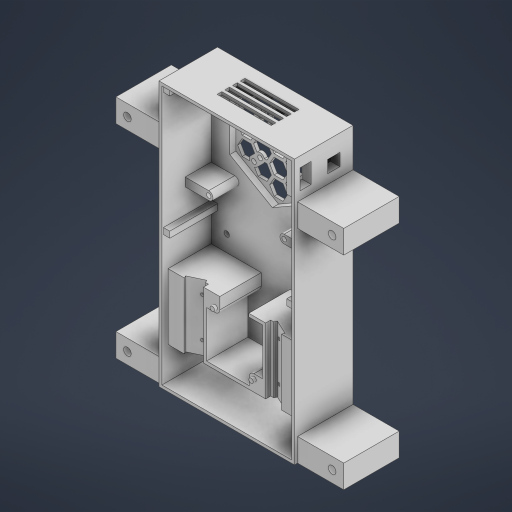
# Autodesk Inventor part: PrimaryCase
Saved by Autodesk Inventor 2023 (Build 270158000, 158)
## iProperties
Created: 2023-12-04
Part Number: PrimaryCase
Material: Generic
Document SubType Name: Modeling
Designer: FizzyApple12
Density: 1 g/cm^3
Appearance: Default
Author: FizzyApple12
Autodesk Inventor part; units mm, degrees
ref_plane "YZ Plane" through (0, 0, 0) normal (1, 0, 0) x (0, 1, 0)
ref_plane "XZ Plane" through (0, 0, 0) normal (0, 1, 0) x (-1, 0, 0)
ref_plane "XY Plane" through (0, 0, 0) normal (0, 0, 1) x (1, 0, 0)
sketch "Sketch1" plane through (0, 0, 0) normal (0, 0, 1) x (1, 0, 0)
  line L0 (0, 0) -> (84, 0)
  line L1 (84, 0) -> (84, -84)
  line L2 (84, -84) -> (0, -84)
  line L3 (0, -84) -> (0, 0)
  line L4 (0, 84) -> (84, 84)
  line L5 (84, 84) -> (84, 0)
  line L6 (84, 0) -> (0, 0) construction
  line L7 (0, 0) -> (0, 84)
  line L8 (-2, 86) -> (86, 86)
  line L9 (86, 86) -> (86, -86)
  line L10 (86, -86) -> (-2, -86)
  line L11 (-2, -86) -> (-2, 86)
  line L12 (-2, 86) -> (86, -86) construction
  line L13 (17, 67) -> (67, 67)
  line L14 (67, 67) -> (67, 17)
  line L15 (67, 17) -> (17, 17)
  line L16 (17, 17) -> (17, 67)
  line L17 (0, 0) -> (84, 84) construction
  line L18 (17, 67) -> (67, 17) construction
  line L19 (0, 2) -> (84, 2)
  point P0 (42, 0)
  point P1 (42, 42)
  point P2 (84, 0)
  dimension "d0" = 84
  dimension "d1" = 84
  dimension "d2" = 84
  dimension "d3" = 84
  dimension "d4" = 88
  dimension "d5" = 172
  dimension "d6" = 50
  dimension "d7" = 50
  dimension "d20" = 2
  constraints: 40 end point, 8 parallel, 5 perpendicular, 4 horizontal, 4 midpoint, 2 point on line
  measures "d0" distance of L1.end L2.end
  measures "d1" distance of L0.end L1.end
  measures "d2" distance of L0.start L5.end
  measures "d3" distance of L4.end L5.end
  measures "d4" distance of L9.end L10.end
  measures "d5" distance of L8.end L9.end
  measures "d6" distance of L14.end L15.end
  measures "d7" distance of L13.end L14.end
  measures "d20" distance between parallel lines of L0 L19
extrude "Extrusion1" add sketch "Sketch1" against normal blind 40 contours L8 L9 L10 L11
sketch "Sketch3" plane through (0, 0, -40) normal (0, 0, -1) x (-1, 0, 0)
  line L0 (2, 86) -> (-86, 86) projected
  line L1 (-86, 86) -> (-86, -86) projected
  line L2 (2, -86) -> (2, 86) projected
  line L3 (-86, -86) -> (2, -86) projected
  point P0 (0, 0)
extrude "Extrusion3" add sketch "Sketch3" against normal blind 8
sketch "Sketch4" plane through (0, 0, -32) normal (0, 0, 1) x (1, 0, 0)
  line L0 (15.1526, 80.5155) -> (64.1526, 80.5155) construction
  line L1 (64.1526, 80.5155) -> (64.1526, 22.5155) construction
  line L2 (64.1526, 22.5155) -> (15.1526, 22.5155) construction
  line L3 (15.1526, 22.5155) -> (15.1526, 80.5155) construction
  line L4 (0, 84) -> (84, 84) construction
  line L5 (0, -84) -> (0, 84) construction
  circle A0 centre (15.1526, 80.5155) radius 2.75
  circle A1 centre (64.1526, 80.5155) radius 2.75
  circle A2 centre (64.1526, 22.5155) radius 2.75
  circle A3 centre (15.1526, 22.5155) radius 2.75
  line L6 (0, 84) -> (17.9026, 84)
  line L7 (17.9026, 84) -> (17.9026, 77.7655)
  line L8 (17.9026, 77.7655) -> (0, 77.7655)
  line L9 (0, 77.7655) -> (0, 84)
  line L10 (84, 84) -> (84, -84) construction
  line L11 (84, 84) -> (61.4026, 84)
  line L12 (61.4026, 84) -> (61.4026, 77.7655)
  line L13 (61.4026, 77.7655) -> (84, 77.7655)
  line L14 (84, 77.7655) -> (84, 84)
  line L15 (84, 25.2655) -> (61.4026, 25.2655)
  line L16 (61.4026, 25.2655) -> (61.4026, 19.7655)
  line L17 (61.4026, 19.7655) -> (84, 19.7655)
  line L18 (84, 19.7655) -> (84, 25.2655)
  line L19 (0, 25.2655) -> (17.9026, 25.2655)
  line L20 (17.9026, 25.2655) -> (17.9026, 19.7655)
  line L21 (17.9026, 19.7655) -> (0, 19.7655)
  line L22 (0, 19.7655) -> (0, 25.2655)
  circle A4 centre (15.1526, 80.5155) radius 1.45
  circle A5 centre (64.1526, 80.5155) radius 1.45
  circle A6 centre (64.1526, 22.5155) radius 1.45
  circle A7 centre (15.1526, 22.5155) radius 1.45
  point P0 (0, 0)
  point P1 (61.4026, 80.5155)
  point P2 (64.1526, 77.7655)
  point P3 (15.1526, 77.7655)
  point P4 (17.9026, 80.5155)
  point P5 (64.1526, 25.2655)
  point P6 (64.1526, 19.7655)
  point P7 (15.1526, 19.7655)
  point P8 (15.1526, 25.2655)
  dimension "d23" = 49
  dimension "d24" = 58
  dimension "d25" = 3.4845
  dimension "d26" = 15.1526
  dimension "d27" = 5.5
  dimension "d30" = 2.9
  constraints: 40 end point, 10 parallel, 9 tangent, 8 centre point, 8 coincident, 6 equal radius, 5 horizontal, 5 perpendicular, 3 point on line
  measures "d23" distance of L1.end L2.end
  measures "d24" distance of L0.end L1.end
  measures "d25" distance between parallel lines of L4 L0
  measures "d26" distance between parallel lines of L5 L3
  measures "d27" diameter of A0
  measures "d30" diameter of A4
extrude "Extrusion4" add sketch "Sketch4" along normal blind 16.86 contours A0 | A0 L8 L9 L6 L7 | A1 | A1 L12 L11 L14 L13 | A2 | A2 L15 L18 L17 | A3 | A3 L21 L22 L19
extrude "Extrusion5" cut sketch "Sketch4" against normal through all contours A4 | A5 | A6 | A7
sketch "Sketch5" plane through (0, 0, -40) normal (0, 0, -1) x (-1, 0, 0)
  circle A0 centre (-15.1526, 80.5155) radius 1.45 construction
  circle A1 centre (-64.1526, 80.5155) radius 1.45 construction
  circle A2 centre (-64.1526, 22.5155) radius 1.45 construction
  circle A3 centre (-15.1526, 22.5155) radius 1.45 construction
  circle A4 centre (-64.1526, 80.5155) radius 2.75
  circle A5 centre (-15.1526, 80.5155) radius 2.75
  circle A6 centre (-15.1526, 22.5155) radius 2.75
  circle A7 centre (-64.1526, 22.5155) radius 2.75
  point P0 (0, 0)
  dimension "d33" = 5.5
  constraints: 4 centre point, 4 coincident, 3 equal radius
  measures "d33" diameter of A4
extrude "Extrusion6" cut sketch "Sketch5" against normal blind 4.86
sketch "Sketch6" plane through (-2, 86, 0) normal (0, -1, 0) x (1, 0, 0)
  line L0 (47.633, -13.54) -> (35.633, -13.54)
  line L1 (35.633, -13.54) -> (35.633, -12.12)
  line L2 (35.633, -12.12) -> (47.633, -12.12)
  line L3 (47.633, -12.12) -> (47.633, -13.54)
  line L4 (2, 0) -> (2, -32) construction
  line L5 (0, 0) -> (88, 0) construction
  line L6 (26.5, -11.33) -> (61.5, -11.33)
  line L7 (61.5, -11.33) -> (61.5, -14.33)
  line L8 (61.5, -14.33) -> (26.5, -14.33)
  line L9 (26.5, -14.33) -> (26.5, -11.33)
  line L10 (44, 0) -> (44, -11.33) construction
  line L11 (88, 0) -> (0, 0) construction
  line L12 (47.633, -12.83) -> (61.5, -12.83) construction
  line L13 (26.5, -19.33) -> (26.5, -16.33)
  line L14 (61.5, -19.33) -> (26.5, -19.33)
  line L15 (26.5, -16.33) -> (61.5, -16.33)
  line L16 (61.5, -16.33) -> (61.5, -19.33)
  line L17 (26.5, -24.33) -> (26.5, -21.33)
  line L18 (61.5, -24.33) -> (26.5, -24.33)
  line L19 (26.5, -21.33) -> (61.5, -21.33)
  line L20 (61.5, -21.33) -> (61.5, -24.33)
  line L21 (26.5, -29.33) -> (26.5, -26.33)
  line L22 (61.5, -29.33) -> (26.5, -29.33)
  line L23 (26.5, -26.33) -> (61.5, -26.33)
  line L24 (61.5, -26.33) -> (61.5, -29.33)
  point P0 (44, -16.33)
  point P1 (61.5, -17.83)
  point P2 (44, -21.33)
  point P3 (61.5, -22.83)
  point P4 (44, -26.33)
  point P5 (61.5, -27.83)
  dimension "d37" = 12
  dimension "d38" = 1.42
  dimension "d39" = 33.633
  dimension "d40" = 12.12
  dimension "d168" = 35
  dimension "d169" = 3
  dimension "d172" = 5
  constraints: 44 end point, 4 midpoint, 4 parallel, 4 perpendicular, 2 horizontal, 1 vertical, 30 other
  measures "d37" distance of L1.end L2.end
  measures "d38" distance of L0.end L1.end
  measures "d39" distance between parallel lines of L1 L4
  measures "d40" distance between parallel lines of L5 L2
  measures "d168" distance of L7.end L8.end
  measures "d169" distance of L6.end L7.end
  measures "d172" distance of L8.end L13.start
extrude "Extrusion7" cut sketch "Sketch6" along normal blind 10 contours L0 L1 L2 L3 | L6 L7 L8 L9 | L13 L15 L16 L14 | L17 L19 L20 L18 | L21 L23 L24 L22
sketch "Sketch7" plane through (0, 0, -32) normal (0, 0, 1) x (1, 0, 0)
  line L0 (0, 84) -> (84, 84) construction
  line L1 (84, 84) -> (0, 84) construction
  line L2 (0, 84) -> (0, 0) construction
  line L3 (0, 0) -> (84, 0) construction
  line L4 (84, 0) -> (84, 84) construction
  line L5 (84, 0) -> (80, 0)
  line L6 (80, 0) -> (80, 4)
  line L7 (80, 4) -> (84, 4)
  line L8 (84, 4) -> (84, 0)
  line L9 (0, 0) -> (4, 0)
  line L10 (4, 0) -> (4, 4)
  line L11 (4, 4) -> (0, 4)
  line L12 (0, 4) -> (0, 0)
  line L13 (0, 84) -> (4, 84)
  line L14 (4, 84) -> (4, 80)
  line L15 (4, 80) -> (0, 80)
  line L16 (0, 80) -> (0, 84)
  line L17 (84, 84) -> (80, 84)
  line L18 (80, 84) -> (80, 77.7655)
  line L19 (80, 77.7655) -> (84, 77.7655)
  line L20 (84, 77.7655) -> (84, 84)
  line L21 (84, 77.7655) -> (64.1526, 77.7655) construction
  point P0 (0, 0)
  dimension "d45" = 84
  dimension "d46" = 84
  dimension "d47" = 4
  dimension "d48" = 4
  constraints: 40 end point, 10 parallel, 5 equal length, 5 horizontal, 5 perpendicular, 1 point on line
  measures "d45" distance of L3.end L2.end
  measures "d46" distance of L2.end L1.end
  measures "d47" distance of L6.end L7.end
  measures "d48" distance of L5.end L6.end
extrude "Extrusion8" add sketch "Sketch7" along normal blind 31
sketch "Sketch8" plane through (0, 0, -32) normal (0, 0, 1) x (1, 0, 0)
  line L0 (21.8, -20.65) -> (62.2, -20.65)
  line L1 (62.2, -20.65) -> (62.2, -63.35)
  line L2 (62.2, -63.35) -> (21.8, -63.35)
  line L3 (21.8, -63.35) -> (21.8, -20.65)
  circle A0 centre (29.4, -28.15) radius 1.45
  circle A1 centre (54.6, -55.95) radius 1.45
  line L4 (21.8, -20.65) -> (62.2, -63.35) construction
  line L5 (84, 0) -> (84, -84) construction
  line L6 (84, -84) -> (0, -84) construction
  line L7 (84, 0) -> (0, -84) construction
  line L8 (23.8, -22.7639) -> (60.2, -22.7639)
  line L9 (60.2, -22.7639) -> (60.2, -61.2361)
  line L10 (60.2, -61.2361) -> (23.8, -61.2361)
  line L11 (23.8, -61.2361) -> (23.8, -22.7639)
  line L12 (23.8, -22.7639) -> (60.2, -61.2361) construction
  line L13 (60.2, -22.7639) -> (23.8, -61.2361) construction
  circle A2 centre (29.4, -28.15) radius 3
  circle A3 centre (54.6, -55.95) radius 3
  line L14 (29.4, -31.15) -> (23.8, -31.15)
  line L15 (32.4, -28.15) -> (32.4, -22.7639)
  line L16 (51.6, -55.95) -> (51.6, -61.2361)
  line L17 (54.6, -52.95) -> (60.2, -52.95)
  line L18 (32.4, -20.65) -> (51.2, -20.65)
  line L19 (51.2, -20.65) -> (51.2, -22.7639)
  line L20 (51.2, -22.7639) -> (32.4, -22.7639)
  line L21 (32.4, -22.7639) -> (32.4, -20.65)
  point P0 (0, 0)
  point P1 (42, -42)
  point P2 (32.4, -22.7639)
  dimension "d51" = 40.4
  dimension "d52" = 42.7
  dimension "d53" = 2.9
  dimension "d54" = 7.6
  dimension "d55" = 7.6
  dimension "d56" = 7.5
  dimension "d57" = 7.4
  dimension "d58" = 2
  dimension "d59" = 6
  dimension "d61" = 11
  constraints: 40 end point, 7 perpendicular, 7 point on line, 6 parallel, 4 centre point, 4 midpoint, 4 point on circle, 4 tangent, 3 horizontal, 2 coincident, 2 equal radius, 1 collinear
  measures "d51" distance of L1.end L2.end
  measures "d52" distance of L0.end L1.end
  measures "d53" diameter of A0
  measures "d54" distance from line of L3 A0.centre
  measures "d55" distance from line of L1 A1.centre
  measures "d56" distance from line of L0 A0.centre
  measures "d57" distance from line of L2 A1.centre
  measures "d58" distance between parallel lines of L1 L9
  measures "d59" diameter of A2
  measures "d61" distance between parallel lines of L1 L19
extrude "Extrusion9" add sketch "Sketch8" along normal blind 27 contours L0 L21 L8 L11 L10 L9 L19 L1 L2 L3 | L15 A2 L14 L11 L8 | A2 | L9 L10 L16 A3 L17 | A3
extrude "Extrusion10" add sketch "Sketch8" along normal blind 28.8 contours A0 | A1
sketch "Sketch9" plane through (21.8, -63.35, -32) normal (0, -1, 0) x (1, 0, 0)
  line L0 (40.4, 0) -> (0, 0) projected
  line L1 (40.4, 0) -> (40.4, 27) projected
  line L2 (0, 27) -> (40.4, 27) projected
  line L3 (0, 0) -> (0, 27) projected
  line L4 (62.2, 0) -> (-21.8, 0) projected
  line L5 (-21.8, 32) -> (-21.8, 0) projected
  line L6 (62.2, 32) -> (-21.8, 32) projected
  line L7 (62.2, 32) -> (62.2, 0) projected
  line L8 (-12.1138, 26.3686) -> (-11.3531, 28)
  line L9 (-11.3531, 28) -> (-2, 23.6386) construction
  line L10 (-2, 23.6386) -> (-2.7607, 22.0072)
  line L11 (-2.7607, 22.0072) -> (-12.1138, 26.3686)
  line L12 (51.7531, 28) -> (42.4, 23.6386) construction
  line L13 (42.4, 23.6386) -> (43.1607, 22.0072)
  line L14 (43.1607, 22.0072) -> (52.5138, 26.3686)
  line L15 (52.5138, 26.3686) -> (51.7531, 28)
  line L16 (-11.3531, 28) -> (51.7531, 28) construction
  line L17 (-21.8, 28) -> (-11.3531, 28)
  line L18 (51.7531, 28) -> (62.2, 28)
  line L19 (-2, 23.6386) -> (0, 23.6386)
  line L20 (42.4, 23.6386) -> (40.4, 23.6386)
  point P0 (-21.8, 32)
  dimension "d66" = 1.8
  dimension "d67" = 10.32
  dimension "d68" = 25
  dimension "d69" = 4
  dimension "d70" = 25
  dimension "d73" = 2
  constraints: 26 end point, 5 parallel, 5 point on line, 3 equal length, 3 perpendicular, 2 collinear
  measures "d66" distance of L8.start L8.end
  measures "d67" distance of L8.end L9.end
  measures "d68" angle of L3 L10
  measures "d69" distance between parallel lines of L6 L16
  measures "d70" angle of L13 L1
  measures "d73" distance of L9.end L19.end
extrude "Extrusion11" add sketch "Sketch9" against normal up to surface (42.7 mm away) contours L1 L20 L13 L14 L15 L18 L7 L4 | L4 L5 L17 L8 L11 L10 L19 L3
sketch "Sketch10" plane through (9.6862, -63.35, -5.6314) normal (0.4226183, 0, 0.9063078) x (0.9063078, 0, -0.4226183)
  line L0 (8.22, 8.5538) -> (8.22, 34.1462) construction
  circle A0 centre (8.22, 8.5538) radius 0.95
  circle A1 centre (8.22, 34.1462) radius 0.95
  line L1 (10.32, 0) -> (10.32, 42.7) construction
  line L2 (10.32, 21.35) -> (8.22, 21.35) construction
  point P0 (-11.1586, 63.35)
  dimension "d74" = 25.5925
  dimension "d75" = 1.9
  dimension "d76" = 2.1
  constraints: 4 end point, 2 centre point, 2 coincident, 2 midpoint, 1 equal radius, 1 perpendicular, 1 vertical
  measures "d74" distance of L0.start L0.end
  measures "d75" diameter of A0
  measures "d76" distance of L2.start L2.end
extrude "Extrusion12" cut sketch "Sketch10" against normal blind 10
sketch "Sketch11" plane through (64.9607, -63.35, -9.9928) normal (-0.4226183, 0, 0.9063078) x (0.9063078, 0, 0.4226183)
  line L0 (2.1, 8.5538) -> (2.1, 34.1462) construction
  line L1 (0, 0) -> (0, 42.7) construction
  line L2 (0, 21.35) -> (2.1, 21.35) construction
  circle A0 centre (2.1, 8.5538) radius 0.95
  circle A1 centre (2.1, 34.1462) radius 0.95
  point P0 (-54.6513, 63.35)
  dimension "d79" = 25.5925
  dimension "d80" = 2.1
  dimension "d81" = 1.9
  constraints: 4 end point, 2 centre point, 2 coincident, 2 midpoint, 1 equal radius, 1 perpendicular, 1 vertical
  measures "d79" distance of L0.start L0.end
  measures "d80" distance of L2.start L2.end
  measures "d81" diameter of A0
extrude "Extrusion13" cut sketch "Sketch11" against normal blind 10
sketch "Sketch13" plane through (0, 0, -32) normal (0, 0, 1) x (1, 0, 0)
  line L0 (84, 77.7655) -> (84, 25.2655) projected
  line L1 (84, 77.7655) -> (80, 77.7655)
  line L2 (80, 77.7655) -> (80, 62.7655)
  line L3 (80, 62.7655) -> (84, 62.7655)
  line L4 (84, 62.7655) -> (84, 77.7655)
  point P0 (0, 0)
  dimension "d93" = 4
  dimension "d94" = 15
  constraints: 8 end point, 2 parallel, 1 horizontal, 1 perpendicular
  measures "d93" distance of L3.end L2.end
  measures "d94" distance of L1.end L2.end
extrude "Extrusion15" add sketch "Sketch13" along normal blind 31
sketch "Sketch12" plane through (86, -86, 0) normal (1, 0, 0) x (0, 0, -1)
  line L0 (8.79, 163.3042) -> (5.63, 163.3042)
  line L1 (5.63, 163.3042) -> (5.63, 154.3642)
  line L2 (5.63, 154.3642) -> (8.79, 154.3642)
  line L3 (8.79, 154.3642) -> (8.79, 163.3042)
  line L4 (0, 0) -> (0, 172) construction
  line L5 (0, 172) -> (40, 172) construction
  line L6 (21.5143, 161.0409) -> (29.5143, 161.0409)
  line L7 (29.5143, 161.0409) -> (29.5143, 153.0409)
  line L8 (29.5143, 153.0409) -> (21.5143, 153.0409)
  line L9 (21.5143, 153.0409) -> (21.5143, 161.0409)
  point P0 (0, 86)
  dimension "d84" = 5.63
  dimension "d85" = 8.79
  dimension "d88" = 8.94
  dimension "d89" = 8.6958
  dimension "d124" = 8
  dimension "d125" = 8
  constraints: 16 end point, 4 parallel, 2 horizontal, 2 perpendicular
  measures "d84" distance between parallel lines of L4 L1
  measures "d85" distance between parallel lines of L4 L3
  measures "d88" distance between parallel lines of L2 L0
  measures "d89" distance between parallel lines of L0 L5
  measures "d124" distance of L7.end L8.end
  measures "d125" distance of L6.end L7.end
extrude "Extrusion14" cut sketch "Sketch12" against normal blind 10
thicken "Thicken2" operation cut thickness 2 both sides no extend neighbours no toward (0, 0, -1) faces at (82, 71.3442, -8.79) (84, 77.3042, -7.7367) (82, 71.3442, -5.63) (84, 68.3642, -6.6833)
thicken "Thicken3" operation cut thickness 0.1 both sides no extend neighbours no toward (1, 0, 0) faces at (84, 50.2655, -16.0467) (36.1667, 84, -4.4433) (0, 36.4218, -5.7133) (56, -84, -10.6667)
sketch "Sketch14" plane through (0, 0, -40) normal (0, 0, -1) x (-1, 0, 0)
  line L0 (-116, -71) -> (-86, -71)
  line L1 (-86, -71) -> (-86, -86)
  line L2 (-86, -86) -> (-116, -86)
  line L3 (-116, -86) -> (-116, -71)
  line L4 (-116, 61) -> (-86, 61)
  line L5 (-86, 61) -> (-86, 46)
  line L6 (-86, 46) -> (-116, 46)
  line L7 (-116, 46) -> (-116, 61)
  line L8 (2, 61) -> (32, 61)
  line L9 (32, 61) -> (32, 46)
  line L10 (32, 46) -> (2, 46)
  line L11 (2, 46) -> (2, 61)
  line L12 (2, -71) -> (32, -71)
  line L13 (32, -71) -> (32, -86)
  line L14 (32, -86) -> (2, -86)
  line L15 (2, -86) -> (2, -71)
  circle A0 centre (-108.5, 53.5) radius 2.45
  line L16 (-116, 61) -> (-101, 46) construction
  line L17 (-116, 61) -> (-94.7868, 61) construction
  line L18 (32, 61) -> (17, 46) construction
  line L19 (32, -86) -> (17, -71) construction
  line L20 (-116, -86) -> (-101, -71) construction
  circle A1 centre (-108.5, -78.5) radius 2.45
  circle A2 centre (24.5, -78.5) radius 2.45
  circle A3 centre (24.5, 53.5) radius 2.45
  line L21 (2, 86) -> (-86, 86) construction
  line L22 (-86, 86) -> (-86, -86) construction
  line L23 (2, -86) -> (2, 86) construction
  point P0 (0, 0)
  dimension "d105" = 30
  dimension "d106" = 15
  dimension "d111" = 4.9
  dimension "d112" = 45
  dimension "d118" = 25
  constraints: 42 end point, 10 equal length, 9 midpoint, 8 parallel, 5 horizontal, 4 centre point, 4 perpendicular, 3 coincident, 3 collinear, 3 equal radius, 1 other
  measures "d105" distance of L5.end L6.end
  measures "d106" distance of L4.end L5.end
  measures "d111" diameter of A0
  measures "d112" angle of L16 L17
extrude "Extrusion16" add sketch "Sketch14" against normal blind 38
extrude "Extrusion17" add sketch "Sketch14" against normal blind 28 contours A0 | A1 | A2 | A3
sketch "Sketch16" plane through (0, 0, -40) normal (0, 0, -1) x (-1, 0, 0)
  line L0 (-55.6526, 67.5155) -> (-23.6526, 67.5155) construction
  line L1 (-23.6526, 67.5155) -> (-23.6526, 35.5155) construction
  line L2 (-23.6526, 35.5155) -> (-55.6526, 35.5155) construction
  line L3 (-55.6526, 35.5155) -> (-55.6526, 67.5155) construction
  line L4 (-55.6526, 67.5155) -> (-23.6526, 35.5155) construction
  line L5 (-23.6526, 67.5155) -> (-55.6526, 35.5155) construction
  line L6 (-51.6526, 63.5155) -> (-27.6526, 63.5155) construction
  line L7 (-27.6526, 63.5155) -> (-27.6526, 39.5155) construction
  line L8 (-27.6526, 39.5155) -> (-51.6526, 39.5155) construction
  line L9 (-51.6526, 39.5155) -> (-51.6526, 63.5155) construction
  line L10 (-51.6526, 63.5155) -> (-27.6526, 39.5155) construction
  line L11 (-27.6526, 63.5155) -> (-51.6526, 39.5155) construction
  circle A0 centre (-55.6526, 67.5155) radius 1.5
  circle A1 centre (-51.6526, 63.5155) radius 1.5
  circle A2 centre (-27.6526, 63.5155) radius 1.5
  circle A3 centre (-23.6526, 67.5155) radius 1.5
  circle A4 centre (-23.6526, 35.5155) radius 1.5
  circle A5 centre (-27.6526, 39.5155) radius 1.5
  circle A6 centre (-55.6526, 35.5155) radius 1.5
  circle A7 centre (-51.6526, 39.5155) radius 1.5
  line L12 (-36.7658, 56.5155) -> (-33.8791, 51.5155)
  line L13 (-33.8791, 51.5155) -> (-36.7658, 46.5155)
  line L14 (-36.7658, 46.5155) -> (-42.5393, 46.5155)
  line L15 (-42.5393, 46.5155) -> (-45.4261, 51.5155)
  line L16 (-45.4261, 51.5155) -> (-42.5393, 56.5155)
  line L17 (-42.5393, 56.5155) -> (-36.7658, 56.5155)
  circle A8 centre (-64.1526, 80.5155) radius 1.45 construction
  circle A9 centre (-15.1526, 22.5155) radius 1.45 construction
  line L18 (-64.1526, 80.5155) -> (-15.1526, 22.5155) construction
  line L19 (-39.6526, 51.5155) -> (-35.3225, 49.0155) construction
  line L20 (-39.6526, 51.5155) -> (-39.6526, 46.5155) construction
  line L21 (-39.6526, 51.5155) -> (-35.3225, 54.0155) construction
  line L22 (-45.4261, 39.5155) -> (-42.5393, 44.5155)
  line L23 (-42.5393, 44.5155) -> (-36.7658, 44.5155)
  line L24 (-36.7658, 44.5155) -> (-33.8791, 39.5155)
  line L25 (-33.8791, 39.5155) -> (-36.7658, 34.5155)
  line L26 (-36.7658, 34.5155) -> (-42.5393, 34.5155)
  line L27 (-42.5393, 34.5155) -> (-45.4261, 39.5155)
  line L28 (-45.4261, 27.5155) -> (-42.5393, 32.5155)
  line L29 (-42.5393, 32.5155) -> (-36.7658, 32.5155)
  line L30 (-36.7658, 32.5155) -> (-33.8791, 27.5155)
  line L31 (-33.8791, 27.5155) -> (-36.7658, 22.5155)
  line L32 (-36.7658, 22.5155) -> (-42.5393, 22.5155)
  line L33 (-42.5393, 22.5155) -> (-45.4261, 27.5155)
  line L34 (-35.0338, 45.5155) -> (-32.147, 50.5155)
  line L35 (-32.147, 40.5155) -> (-35.0338, 45.5155)
  line L36 (-32.147, 50.5155) -> (-26.3735, 50.5155)
  line L37 (-26.3735, 50.5155) -> (-23.4868, 45.5155)
  line L38 (-23.4868, 45.5155) -> (-26.3735, 40.5155)
  line L39 (-26.3735, 40.5155) -> (-32.147, 40.5155)
  line L40 (-21.7547, 34.5155) -> (-24.6415, 39.5155)
  line L41 (-24.6415, 39.5155) -> (-21.7547, 44.5155)
  line L42 (-15.9812, 34.5155) -> (-21.7547, 34.5155)
  line L43 (-13.0945, 39.5155) -> (-15.9812, 34.5155)
  line L44 (-15.9812, 44.5155) -> (-13.0945, 39.5155)
  line L45 (-21.7547, 44.5155) -> (-15.9812, 44.5155)
  line L46 (-32.147, 52.5155) -> (-35.0338, 57.5155)
  line L47 (-26.3735, 52.5155) -> (-32.147, 52.5155)
  line L48 (-35.0338, 57.5155) -> (-32.147, 62.5155)
  line L49 (-32.147, 62.5155) -> (-26.3735, 62.5155)
  line L50 (-26.3735, 62.5155) -> (-23.4868, 57.5155)
  line L51 (-23.4868, 57.5155) -> (-26.3735, 52.5155)
  line L52 (-15.9812, 58.5155) -> (-21.7547, 58.5155)
  line L53 (-21.7547, 58.5155) -> (-24.6415, 63.5155)
  line L54 (-13.0945, 63.5155) -> (-15.9812, 58.5155)
  line L55 (-15.9812, 68.5155) -> (-13.0945, 63.5155)
  line L56 (-21.7547, 68.5155) -> (-15.9812, 68.5155)
  line L57 (-24.6415, 63.5155) -> (-21.7547, 68.5155)
  line L58 (-36.7658, 58.5155) -> (-42.5393, 58.5155)
  line L59 (-33.8791, 63.5155) -> (-36.7658, 58.5155)
  line L60 (-42.5393, 58.5155) -> (-45.4261, 63.5155)
  line L61 (-45.4261, 63.5155) -> (-42.5393, 68.5155)
  line L62 (-42.5393, 68.5155) -> (-36.7658, 68.5155)
  line L63 (-36.7658, 68.5155) -> (-33.8791, 63.5155)
  line L64 (-33.8791, 75.5155) -> (-36.7658, 70.5155)
  line L65 (-36.7658, 70.5155) -> (-42.5393, 70.5155)
  line L66 (-36.7658, 80.5155) -> (-33.8791, 75.5155)
  line L67 (-42.5393, 80.5155) -> (-36.7658, 80.5155)
  line L68 (-45.4261, 75.5155) -> (-42.5393, 80.5155)
  line L69 (-42.5393, 70.5155) -> (-45.4261, 75.5155)
  line L70 (-44.2714, 57.5155) -> (-47.1581, 52.5155)
  line L71 (-47.1581, 62.5155) -> (-44.2714, 57.5155)
  line L72 (-47.1581, 52.5155) -> (-52.9316, 52.5155)
  line L73 (-52.9316, 52.5155) -> (-55.8184, 57.5155)
  line L74 (-55.8184, 57.5155) -> (-52.9316, 62.5155)
  line L75 (-52.9316, 62.5155) -> (-47.1581, 62.5155)
  line L76 (-57.5504, 68.5155) -> (-54.6637, 63.5155)
  line L77 (-54.6637, 63.5155) -> (-57.5504, 58.5155)
  line L78 (-63.3239, 68.5155) -> (-57.5504, 68.5155)
  line L79 (-66.2107, 63.5155) -> (-63.3239, 68.5155)
  line L80 (-63.3239, 58.5155) -> (-66.2107, 63.5155)
  line L81 (-57.5504, 58.5155) -> (-63.3239, 58.5155)
  line L82 (-47.1581, 50.5155) -> (-44.2714, 45.5155)
  line L83 (-52.9316, 50.5155) -> (-47.1581, 50.5155)
  line L84 (-44.2714, 45.5155) -> (-47.1581, 40.5155)
  line L85 (-47.1581, 40.5155) -> (-52.9316, 40.5155)
  line L86 (-52.9316, 40.5155) -> (-55.8184, 45.5155)
  line L87 (-55.8184, 45.5155) -> (-52.9316, 50.5155)
  line L88 (-63.3239, 44.5155) -> (-57.5504, 44.5155)
  line L89 (-57.5504, 44.5155) -> (-54.6637, 39.5155)
  line L90 (-66.2107, 39.5155) -> (-63.3239, 44.5155)
  line L91 (-63.3239, 34.5155) -> (-66.2107, 39.5155)
  line L92 (-57.5504, 34.5155) -> (-63.3239, 34.5155)
  line L93 (-54.6637, 39.5155) -> (-57.5504, 34.5155)
  line L94 (-44.2714, 33.5155) -> (-47.1581, 28.5155)
  line L95 (-47.1581, 38.5155) -> (-44.2714, 33.5155)
  line L96 (-52.9316, 38.5155) -> (-47.1581, 38.5155)
  line L97 (-55.8184, 33.5155) -> (-52.9316, 38.5155)
  line L98 (-52.9316, 28.5155) -> (-55.8184, 33.5155)
  line L99 (-47.1581, 28.5155) -> (-52.9316, 28.5155)
  line L100 (-26.3735, 64.5155) -> (-32.147, 64.5155)
  line L101 (-32.147, 64.5155) -> (-35.0338, 69.5155)
  line L102 (-35.0338, 69.5155) -> (-32.147, 74.5155)
  line L103 (-32.147, 74.5155) -> (-26.3735, 74.5155)
  line L104 (-26.3735, 74.5155) -> (-23.4868, 69.5155)
  line L105 (-23.4868, 69.5155) -> (-26.3735, 64.5155)
  line L106 (-15.9812, 46.5155) -> (-21.7547, 46.5155)
  line L107 (-21.7547, 46.5155) -> (-24.6415, 51.5155)
  line L108 (-24.6415, 51.5155) -> (-21.7547, 56.5155)
  line L109 (-21.7547, 56.5155) -> (-15.9812, 56.5155)
  line L110 (-13.0945, 51.5155) -> (-15.9812, 46.5155)
  line L111 (-15.9812, 56.5155) -> (-13.0945, 51.5155)
  line L112 (-26.3735, 28.5155) -> (-32.147, 28.5155)
  line L113 (-32.147, 28.5155) -> (-35.0338, 33.5155)
  line L114 (-35.0338, 33.5155) -> (-32.147, 38.5155)
  line L115 (-32.147, 38.5155) -> (-26.3735, 38.5155)
  line L116 (-26.3735, 38.5155) -> (-23.4868, 33.5155)
  line L117 (-23.4868, 33.5155) -> (-26.3735, 28.5155)
  line L118 (-66.2107, 51.5155) -> (-63.3239, 56.5155)
  line L119 (-63.3239, 46.5155) -> (-66.2107, 51.5155)
  line L120 (-57.5504, 46.5155) -> (-63.3239, 46.5155)
  line L121 (-54.6637, 51.5155) -> (-57.5504, 46.5155)
  line L122 (-57.5504, 56.5155) -> (-54.6637, 51.5155)
  line L123 (-63.3239, 56.5155) -> (-57.5504, 56.5155)
  line L124 (-52.9316, 64.5155) -> (-55.8184, 69.5155)
  line L125 (-55.8184, 69.5155) -> (-52.9316, 74.5155)
  line L126 (-52.9316, 74.5155) -> (-47.1581, 74.5155)
  line L127 (-47.1581, 74.5155) -> (-44.2714, 69.5155)
  line L128 (-44.2714, 69.5155) -> (-47.1581, 64.5155)
  line L129 (-47.1581, 64.5155) -> (-52.9316, 64.5155)
  line L130 (-55.6526, 67.5155) -> (-51.6526, 63.5155) construction
  line L131 (-57.7739, 65.3942) -> (-53.7739, 61.3942)
  line L132 (-49.5313, 65.6369) -> (-53.5313, 69.6369)
  arc A10 (-53.5313, 69.6369) -> (-57.7739, 65.3942) centre (-55.6526, 67.5155) ccw
  arc A11 (-53.7739, 61.3942) -> (-49.5313, 65.6369) centre (-51.6526, 63.5155) ccw
  line L133 (-23.6526, 67.5155) -> (-27.6526, 63.5155) construction
  line L134 (-25.7739, 69.6369) -> (-29.7739, 65.6369)
  line L135 (-25.5313, 61.3942) -> (-21.5313, 65.3942)
  arc A12 (-21.5313, 65.3942) -> (-25.7739, 69.6369) centre (-23.6526, 67.5155) ccw
  arc A13 (-29.7739, 65.6369) -> (-25.5313, 61.3942) centre (-27.6526, 63.5155) ccw
  line L136 (-23.6526, 35.5155) -> (-27.6526, 39.5155) construction
  line L137 (-21.5313, 37.6369) -> (-25.5313, 41.6369)
  line L138 (-29.7739, 37.3942) -> (-25.7739, 33.3942)
  arc A14 (-25.7739, 33.3942) -> (-21.5313, 37.6369) centre (-23.6526, 35.5155) ccw
  arc A15 (-25.5313, 41.6369) -> (-29.7739, 37.3942) centre (-27.6526, 39.5155) ccw
  line L139 (-51.6526, 39.5155) -> (-55.6526, 35.5155) construction
  line L140 (-53.7739, 41.6369) -> (-57.7739, 37.6369)
  line L141 (-53.5313, 33.3942) -> (-49.5313, 37.3942)
  arc A16 (-49.5313, 37.3942) -> (-53.7739, 41.6369) centre (-51.6526, 39.5155) ccw
  arc A17 (-57.7739, 37.6369) -> (-53.5313, 33.3942) centre (-55.6526, 35.5155) ccw
  point P0 (0, 0)
  point P1 (-35.3225, 42.0155)
  point P2 (-35.3225, 37.0155)
  point P3 (-39.6526, 34.5155)
  point P4 (-35.3225, 30.0155)
  point P5 (-35.3225, 25.0155)
  point P6 (-39.6526, 22.5155)
  point P7 (-29.2603, 50.5155)
  point P8 (-24.9301, 48.0155)
  point P9 (-24.9301, 43.0155)
  point P10 (-14.5378, 37.0155)
  point P11 (-14.5378, 42.0155)
  point P12 (-18.868, 44.5155)
  point P13 (-33.5904, 60.0155)
  point P14 (-29.2603, 62.5155)
  point P15 (-24.9301, 60.0155)
  point P16 (-14.5378, 66.0155)
  point P17 (-18.868, 68.5155)
  point P18 (-23.1981, 66.0155)
  point P19 (-43.9827, 61.0155)
  point P20 (-43.9827, 66.0155)
  point P21 (-39.6526, 68.5155)
  point P22 (-39.6526, 80.5155)
  point P23 (-43.9827, 78.0155)
  point P24 (-43.9827, 73.0155)
  point P25 (-50.0449, 52.5155)
  point P26 (-54.375, 55.0155)
  point P27 (-54.375, 60.0155)
  point P28 (-64.7673, 66.0155)
  point P29 (-64.7673, 61.0155)
  point P30 (-60.4372, 58.5155)
  point P31 (-45.7148, 43.0155)
  point P32 (-50.0449, 40.5155)
  point P33 (-54.375, 43.0155)
  point P34 (-64.7673, 37.0155)
  point P35 (-60.4372, 34.5155)
  point P36 (-56.1071, 37.0155)
  point P37 (-45.7148, 31.0155)
  point P38 (-54.375, 31.0155)
  point P39 (-50.0449, 28.5155)
  point P40 (-33.5904, 67.0155)
  point P41 (-33.5904, 72.0155)
  point P42 (-29.2603, 74.5155)
  point P43 (-23.1981, 54.0155)
  point P44 (-18.868, 56.5155)
  point P45 (-14.5378, 54.0155)
  point P46 (-29.2603, 28.5155)
  point P47 (-24.9301, 36.0155)
  point P48 (-24.9301, 31.0155)
  point P49 (-64.7673, 49.0155)
  point P50 (-60.4372, 46.5155)
  point P51 (-56.1071, 49.0155)
  point P52 (-54.375, 67.0155)
  point P53 (-54.375, 72.0155)
  point P54 (-50.0449, 74.5155)
  point P55 (-53.6526, 65.5155)
  point P56 (-25.6526, 65.5155)
  point P57 (-25.6526, 37.5155)
  point P58 (-53.6526, 37.5155)
  point P59 (-24.0489, 32.5418)
  point P60 (-30.481, 38.5155)
  point P61 (-24.1907, 40.2963)
  point P62 (-20.8242, 34.5155)
  point P63 (-30.481, 40.5155)
  point P64 (-25.6574, 41.7559)
  point P65 (-25.6574, 61.2752)
  point P66 (-30.481, 62.5155)
  point P67 (-20.8242, 68.5155)
  point P68 (-24.1907, 62.7348)
  point P69 (-30.481, 64.5155)
  point P70 (-24.0489, 70.4892)
  point P71 (-48.8242, 38.5155)
  point P72 (-55.2562, 32.5418)
  point P73 (-53.6478, 41.7559)
  point P74 (-48.8242, 40.5155)
  point P75 (-58.481, 34.5155)
  point P76 (-55.1145, 40.2963)
  point P77 (-48.8242, 62.5155)
  point P78 (-53.6478, 61.2752)
  point P79 (-55.1145, 62.7348)
  point P80 (-58.481, 68.5155)
  point P81 (-55.2562, 70.4892)
  point P82 (-48.8242, 64.5155)
  dimension "d126" = 32
  dimension "d127" = 32
  dimension "d128" = 24
  dimension "d129" = 24
  dimension "d130" = 3
  dimension "d131" = 10
  dimension "d134" = 12
  dimension "d141" = 360
  dimension "d145" = 12
  dimension "d152" = 12
  dimension "d157" = 6
  dimension "d158" = 6
  dimension "d159" = 6
  dimension "d160" = 6
  constraints: 292 end point, 16 centre point, 16 point on circle, 16 tangent, 12 midpoint, 9 coincident, 8 parallel, 7 equal radius, 3 horizontal, 2 perpendicular, 1 vertical, 316 other
  measures "d126" distance of L1.end L2.end
  measures "d127" distance of L0.end L1.end
  measures "d128" distance of L7.end L8.end
  measures "d129" distance of L6.end L7.end
  measures "d130" diameter of A0
  measures "d131" distance between parallel lines of L14 L17
  measures "d134" distance of L15.end L22.start
  measures "d145" distance of L89.end L94.start
  measures "d152" distance of L86.end L118.start
  measures "d157" diameter of A11
  measures "d158" diameter of A13
  measures "d159" diameter of A15
  measures "d160" diameter of A17
extrude "Extrusion19" cut sketch "Sketch16" against normal blind 10 contours A0 L124 | L124 A0 L76 | L76 A0 | L125 L126 L127 L128 L129 A11 L132 A10 | L129 A1 L75 | A1 L129 | A10 L131 L77 L81 L80 L79 L78 | L75 A1 | A11 L75 L71 L70 L72 L73 L74 | A2 L49 L100 | L100 A2 | A2 L49 | L100 L101 L102 L103 L104 A12 L134 A13 | L105 A3 L57 | A3 L105 | A13 L50 L51 L47 L46 L48 L49 | L57 A3 | L135 A12 L56 L55 L54 L52 L53 | A4 L40 | L40 A4 L116 | L116 A4 | L41 L45 L44 L43 L42 A14 L137 | L115 A5 L39 | A5 L115 | L117 L112 L113 L114 L115 A15 L138 A14 | A15 L39 L35 L34 L36 L37 L38 | A5 L39 | A6 L97 | L97 A6 L93 | L93 A6 | L96 A7 | A7 L85 L96 | A17 L141 A16 L96 L95 L94 L99 L98 | L140 A17 L92 L91 L90 L88 L89 | A7 L85 | L86 L87 L83 L82 L84 L85 A16 | L12 L13 L14 L15 L16 L17 | L22 L23 L24 L25 L26 L27 | L28 L29 L30 L31 L32 L33 | L58 L60 L61 L62 L63 L59 | L64 L65 L69 L68 L67 L66 | L106 L107 L108 L109 L111 L110 | L118 L123 L122 L121 L120 L119
sketch "Sketch17" plane through (0, 0, -40) normal (0, 0, -1) x (-1, 0, 0)
  line L0 (-162.9977, 133.9544) -> (60.4573, 133.9544)
  line L1 (60.4573, 133.9544) -> (60.4573, -126.8418)
  line L2 (60.4573, -126.8418) -> (-162.9977, -126.8418)
  line L3 (-162.9977, -126.8418) -> (-162.9977, 133.9544)
  point P0 (0, 0)
  constraints: 8 end point, 2 parallel, 1 horizontal, 1 perpendicular
extrude "Extrusion20" cut sketch "Sketch17" against normal blind 2
sketch "Sketch18" plane through (0, 0, -32) normal (0, 0, 1) x (1, 0, 0)
  line L0 (42.5393, 46.5155) -> (36.7658, 46.5155) construction
  line L1 (36.7658, 56.5155) -> (42.5393, 56.5155) construction
  line L2 (36.7658, 46.5155) -> (42.5393, 56.5155) construction
  line L3 (39.6526, 83.5155) -> (67.3654, 67.5155)
  line L4 (67.3654, 67.5155) -> (67.3654, 35.5155)
  line L5 (67.3654, 35.5155) -> (39.6526, 19.5155)
  line L6 (39.6526, 19.5155) -> (11.9398, 35.5155)
  line L7 (11.9398, 35.5155) -> (11.9398, 67.5155)
  line L8 (11.9398, 67.5155) -> (39.6526, 83.5155)
  line L9 (39.6526, 83.5155) -> (39.6526, 51.5155) construction
  point P0 (0, 0)
  dimension "d165" = 32
  constraints: 16 end point, 1 midpoint, 1 vertical, 13 other
  measures "d165" distance of L3.start L9.end
extrude "Extrusion21" cut sketch "Sketch18" against normal blind 4
sketch "Sketch20" plane through (0, 0, -38) normal (0, 0, -1) x (-1, 0, 0)
  line L0 (-74, -10.05) -> (-10, -10.05) construction
  line L1 (-10, -10.05) -> (-10, -74.05) construction
  line L2 (-10, -74.05) -> (-74, -74.05) construction
  line L3 (-74, -74.05) -> (-74, -10.05) construction
  line L4 (-10, -10.05) -> (-74, -74.05) construction
  line L5 (-84.1, 0) -> (0.1, -84.1) construction
  point P0 (0, 0)
  point P1 (0.1, -84.1)
  point P2 (-42, -42.05)
  dimension "d177" = 64
  dimension "d178" = 64
  constraints: 12 end point, 6 coincident, 2 midpoint, 2 parallel, 1 horizontal, 1 perpendicular
  measures "d177" distance of L1.end L2.end
  measures "d178" distance of L0.end L1.end
hole "Hole1" at (74, -10.05, -38) at (10, -10.05, -38) at (10, -74.05, -38) at (74, -74.05, -38) direction (0, 0, 1) diameter 3.4 end through all counterbore diameter 6.5 counterbore depth 3 clearance for "Socket Head Cap Screw" size "M3" standard "Ansi Metric M Profile"
fillet "Fillet5" [suppressed]
fillet "Fillet3" [suppressed]
fillet "Fillet4" [suppressed]
chamfer "Chamfer1" [suppressed]
thicken "Thicken4" operation cut thickness 0.1 both sides no extend neighbours no toward (0, 0, -1) faces at (61.5333, -45.65, -5)
equation "\"d70\" = d68"
body "Solid1"
